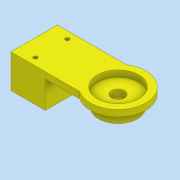
# Autodesk Inventor part: encoder in 6809_ab
Saved by Autodesk Inventor 2020.2 (Build 242310000, 310)
## iProperties
Created: 2016-12-03
Part Number: encoder in 6809_ab
Material: Allgemein
Document SubType Name: Modeling
Designer: paulg
Density: 1 g/cm^3
Appearance: Vorgabe
Author: paulg
Autodesk Inventor part; units mm, degrees
ref_plane "YZ Plane" through (0, 0, 0) normal (1, 0, 0) x (0, 1, 0)
ref_plane "XZ Plane" through (0, 0, 0) normal (0, 1, 0) x (-1, 0, 0)
ref_plane "XY Plane" through (0, 0, 0) normal (0, 0, 1) x (1, 0, 0)
sketch "Sketch1" plane through (0, 0, 0) normal (0, 0, 1) x (1, 0, 0)
  circle A0 centre (0, 0) radius 15.1
  circle A1 centre (0, 0) radius 5
  dimension "d0" = 30.2
  dimension "d1" = 10
  constraints: 2 centre point, 2 coincident
  measures "d0" diameter of A0
  measures "d1" diameter of A1
extrude "Extrusion1" add sketch "Sketch1" along normal blind 8
sketch "Sketch3" plane through (0, 0, 8) normal (0, 0, 1) x (1, 0, 0)
  circle A0 centre (0, 0) radius 5 projected
  circle A1 centre (0, 0) radius 15.1 projected
  circle A2 centre (0, 0) radius 16.1
  dimension "d21" = 1
  constraints: 1 centre point, 1 coincident
  measures "d21" radial gap between concentric circles of A1 A2
extrude "Extrusion3" add sketch "Sketch3" along normal blind 1 contours A1 | A2
sketch "Sketch4" plane through (0, 0, 9) normal (0, 0, 1) x (1, 0, 0)
  circle A0 centre (0, 0) radius 5 projected
  circle A1 centre (0, 0) radius 16.1 projected
  arc A2 (-21.5, 0) -> (-11.758, -18) centre (0, 0) ccw construction
  line L0 (0, 0) -> (-37.0387, 0) construction
  line L1 (-11.758, 18) -> (-65, 18)
  line L2 (-65, 18) -> (-65, -18)
  arc A3 (-65, -18) -> (-65, -18) centre (-67.4575, -18) ccw
  circle A4 centre (-51.6895, 12.375) radius 1.5
  circle A5 centre (-51.6895, -12.375) radius 1.5
  circle A6 centre (0, 0) radius 6
  circle A7 centre (0, 0) radius 9
  line L3 (-65, -18) -> (-11.758, -18)
  line L4 (-11.758, 18) -> (-11.758, -18) construction
  line L5 (-38.379, 18) -> (-38.379, -18)
  line L6 (-51.6895, 12.375) -> (-51.6895, -12.375) construction
  arc A8 (-11.758, 18) -> (-21.5, 0) centre (0, 0) ccw construction
  arc A9 (-11.758, -18) -> (-11.758, 18) centre (0, 0) ccw
  dimension "d22" = 43
  dimension "d31" = 65
  dimension "d623" = 3
  dimension "d624" = 24.75
  dimension "d627" = 12
  dimension "d628" = 3
  dimension "d633" = 36
  constraints: 14 end point, 8 centre point, 8 point on circle, 5 coincident, 3 midpoint, 2 perpendicular, 2 point on line, 2 vertical, 1 equal radius, 1 horizontal, 1 symmetric about line, 1 tangent, 1 other
  measures "d22" diameter of A2
  measures "d31" distance from line of A0.centre L2
  measures "d623" diameter of A4
  measures "d624" distance of A5.centre A4.centre
  measures "d627" diameter of A6
  measures "d628" radial gap between concentric circles of A7 A6
  measures "d633" distance of L2.end L1.end
extrude "Extrusion5" add sketch "Sketch4" along normal blind 5 contours A9 L3 L5 L1 | L5 L3 L2 L1
sketch "Sketch17" plane through (0, 0, 0) normal (0, 0, -1) x (-1, 0, 0)
  circle A0 centre (0, 0) radius 5 projected
  circle A1 centre (0, 0) radius 15.1 projected
  line L0 (0, 0) -> (0, -15.1) construction
  circle A2 centre (0, 0) radius 15.1 projected
  line L1 (0, 0) -> (-5.7785, -13.9506) construction
  circle A3 centre (-4.4965, -10.8556) radius 1.5
  dimension "d100" = 22.5
  dimension "d101" = 3
  dimension "d102" = 11.75
  constraints: 4 end point, 4 point on circle, 1 centre point, 1 point on line, 1 vertical
  measures "d100" angle of L1 L0
  measures "d101" diameter of A3
  measures "d102" distance of A0.centre A3.centre
extrude "Extrusion14" cut sketch "Sketch17" against normal blind 8 contours A3
pattern_circular "Circular Pattern3" count 8 over 360 about axis through (0, 0, 0) along (0, 0, 1) of "Extrusion14"
extrude "Extrusion85" add sketch "Sketch4" against normal blind 21 contours L5 L3 L2 L1
extrude "Extrusion86" cut sketch "Sketch4" along normal through all both and the other way through all contours A4 | A5
extrude "Extrusion88" cut sketch "Sketch4" along normal blind 4 from surface at -9 contours A0 | A6
equation "\"E_\" = 1"
equation "\"Rr_\" = 2"
equation "\"R_\" = 19"
equation "\"Ri\" = 11.75"
equation "\"Ra\" = 21.5"
equation "\"Rl\" = 17.5"
equation "\"Rla\" = 18.5"
equation "\"Rli\" = 15"
equation "\"Rsi\" = 5"
equation "\"Rsa\" = 7.5"
equation "\"Rca\" = 7"
equation "\"Ras\" = 1"
equation "\"Rci\" = 5"
equation "\"Rea\" = 3.5"
equation "\"Rei\" = 2"
body "Solid1"
